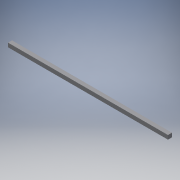
# Autodesk Inventor part: Part89
Saved by Autodesk Inventor 2016 (Build 200138000, 138)
## iProperties
Created: 2016-09-04
Part Number: Part89
Material: Generic
Document SubType Name: Modeling
Designer: gus
Density: 1 g/cm^3
Appearance: Default
Author: gus
Autodesk Inventor part; units mm, degrees
ref_plane "YZ Plane" through (0, 0, 0) normal (1, 0, 0) x (0, 1, 0)
ref_plane "XZ Plane" through (0, 0, 0) normal (0, 1, 0) x (-1, 0, 0)
ref_plane "XY Plane" through (0, 0, 0) normal (0, 0, 1) x (1, 0, 0)
sketch "Sketch1" plane through (0, 0, 0) normal (1, 0, 0) x (0, 1, 0)
  line L0 (0, 0) -> (25.4, 0)
  line L1 (25.4, 0) -> (25.4, 25.4)
  line L2 (25.4, 25.4) -> (0, 25.4)
  line L3 (0, 25.4) -> (0, 0)
  dimension "d0" = 25.4
  dimension "d1" = 25.4
  constraints: 8 end point, 2 parallel, 1 horizontal, 1 perpendicular
  measures "d0" distance of L2.end L1.end
  measures "d1" distance of L1.end L0.end
extrude "Extrusion1" add sketch "Sketch1" along normal blind 838.2
sketch "Sketch2" plane through (0, 0, 25.4) normal (0, 0, 1) x (1, 0, 0)
  circle A0 centre (12.7, 12.7) radius 6.35
  line L0 (0, 25.4) -> (838.2, 25.4) projected
  line L1 (0, 0) -> (0, 25.4) projected
  circle A1 centre (825.5, 12.7) radius 6.35
  line L2 (838.2, 25.4) -> (838.2, 0) projected
  circle A2 centre (153.9916, 12.7) radius 6.35
  dimension "d4" = 12.7
  dimension "d5" = 12.7
  dimension "d6" = 12.7
  dimension "d9" = 12.7
  dimension "d10" = 12.7
  dimension "d11" = 12.7
  dimension "d24" = 12.7
  dimension "d25" = 12.7
  dimension "d26" = 153.9916
  constraints: 3 centre point
  measures "d4" diameter of A0
  measures "d5" distance from line of L0 A0.centre
  measures "d6" distance from line of L1 A0.centre
  measures "d9" diameter of A1
  measures "d10" distance from line of L0 A1.centre
  measures "d11" distance from line of L2 A1.centre
  measures "d24" diameter of A2
  measures "d25" distance from line of A2.centre L0
  measures "d26" distance from line of L1 A2.centre
extrude "Extrusion2" cut sketch "Sketch2" against normal blind 1016
body "Solid1"
